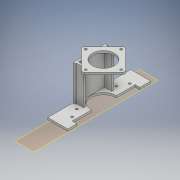
# Autodesk Inventor part: BAseSupport
Saved by Autodesk Inventor 2018 (Build 220112000, 112)
## iProperties
Created: 2017-08-08
Part Number: BAseSupport
Material: Generic
Document SubType Name: Modeling
Designer: M215104
Density: 1 g/cm^3
Appearance: Default
Author: M215104
Autodesk Inventor part; units mm, degrees
ref_plane "YZ Plane" through (0, 0, 0) normal (1, 0, 0) x (0, 1, 0)
ref_plane "XZ Plane" through (0, 0, 0) normal (0, 1, 0) x (-1, 0, 0)
ref_plane "XY Plane" through (0, 0, 0) normal (0, 0, 1) x (1, 0, 0)
ref_plane "Work Plane1" through (0, 2.2013, 0) normal (0, 0, 1) x (1, 0, 0)
sketch "Sketch1" plane through (0, 2.2013, 0) normal (0, 0, 1) x (1, 0, 0)
  arc A0 (50.7, -89.2086) -> (50.7, -149.194) centre (33.15, -119.2013) ccw construction
  circle A1 centre (30.5, -119.2013) radius 14.9 construction
  line L0 (34, -32.2013) -> (47, -32.2013) projected
  line L1 (47, -2.2013) -> (47, -32.2013) construction
  line L2 (0, -2.2013) -> (47, -2.2013) construction
  line L3 (0, -2.2013) -> (0, -315.2013) construction
  line L4 (0, -315.2013) -> (47, -315.2013) construction
  line L5 (47, -207.2013) -> (47, -315.2013) construction
  line L6 (47, -207.2013) -> (34, -207.2013) projected
  line L7 (34, -207.2013) -> (34, -193.2013) construction
  line L8 (34, -193.2013) -> (36, -193.2013) construction
  line L9 (36, -193.2013) -> (36, -155.499) construction
  line L10 (36, -155.499) -> (47, -163.2013) construction
  line L11 (47, -67.2013) -> (47, -163.2013) construction
  line L12 (47, -67.2013) -> (36, -74.9036) construction
  line L13 (36, -74.9036) -> (36, -45.2013) construction
  line L14 (36, -45.2013) -> (34, -45.2013) construction
  line L15 (34, -45.2013) -> (34, -32.2013) construction
  line L16 (47, -32.2013) -> (47, -2.2013)
  line L17 (47, -2.2013) -> (-8, -2.2013)
  line L18 (-8, -2.2013) -> (-8, -232.2013)
  line L19 (-8, -232.2013) -> (47, -232.2013)
  line L20 (47, -207.2013) -> (34, -207.2013) construction
  line L21 (34, -32.2013) -> (47, -32.2013) construction
  line L22 (47, -232.2013) -> (47, -207.2013)
  line L23 (47, -32.2013) -> (34, -32.2013)
  arc A2 (34, -84.4617) -> (34, -153.9409) centre (33.15, -119.2013) ccw
  line L24 (34, -207.2013) -> (34, -153.9409)
  line L25 (34, -84.4617) -> (34, -32.2013)
  dimension "d0" = 55
  dimension "d1" = 230
  constraints: 20 end point, 5 collinear, 2 parallel, 2 perpendicular, 2 point on circle, 2 point on line, 1 centre point, 1 coincident, 1 concentric
  measures "d0" distance of L1.start L17.end
  measures "d1" distance of L17.end L18.end
extrude "Extrusion1" add sketch "Sketch1" along normal blind 6
sketch "Sketch2" plane through (0, 2.2013, 6) normal (0, 0, 1) x (1, 0, 0)
  line L0 (-8, -2.2013) -> (-8, -232.2013) projected
  line L1 (-8, -117.2013) -> (-2, -117.2013)
  line L2 (-2, -117.2013) -> (-2, -162.2013)
  line L3 (-2, -162.2013) -> (-8, -162.2013)
  line L4 (-8, -162.2013) -> (-8, -117.2013)
  line L5 (-2, -117.2013) -> (-2, -72.2013)
  line L6 (-2, -72.2013) -> (-8, -72.2013)
  line L7 (-8, -72.2013) -> (-8, -117.2013)
  point P0 (0, -2.2013)
  dimension "d4" = 6
  dimension "d5" = 45
  constraints: 14 end point, 2 parallel, 2 symmetric about line, 1 horizontal, 1 midpoint, 1 perpendicular
  measures "d4" distance of L2.end L3.end
  measures "d5" distance of L1.end L2.end
extrude "Extrusion2" add sketch "Sketch2" along normal blind 97.5
sketch "Sketch3" plane through (0, 2.2013, 103.5) normal (0, 0, 1) x (1, 0, 0)
  line L0 (34, -207.2013) -> (34, -153.9409) construction
  line L1 (-27.6612, -119.2013) -> (33.15, -58.3901)
  line L2 (33.15, -58.3901) -> (93.9612, -119.2013)
  line L3 (93.9612, -119.2013) -> (33.15, -180.0125)
  line L4 (33.15, -180.0125) -> (-27.6612, -119.2013)
  arc A0 (34, -84.4617) -> (34, -153.9409) centre (33.15, -119.2013) ccw construction
  line L5 (-9.85, -76.2013) -> (76.15, -162.2013) construction
  line L6 (76.15, -76.2013) -> (-9.85, -162.2013) construction
  line L7 (-8, -162.2013) -> (-2, -162.2013) projected
  line L8 (-2, -162.2013) -> (15.3388, -162.2013)
  line L9 (-2, -162.2013) -> (-2, -72.2013) projected
  line L10 (-2, -72.2013) -> (19.3388, -72.2013)
  point P0 (0, -2.2013)
  point P1 (33.15, -117)
  dimension "d8" = 86
  dimension "d9" = 86
  constraints: 16 end point, 2 midpoint, 2 parallel, 2 point on line, 1 collinear, 1 horizontal, 1 perpendicular, 1 other
  measures "d8" distance of L2.end L3.end
  measures "d9" distance of L1.end L2.end
extrude "Extrusion3" add sketch "Sketch3" along normal blind 6 contours L1 L2 L3 L4 L9 | L9 L4 L1
sketch "Sketch4" plane through (0, 2.2013, 109.5) normal (0, 0, 1) x (1, 0, 0)
  arc A0 (34, -84.4617) -> (34, -153.9409) centre (33.15, -119.2013) ccw projected
  circle A1 centre (33.15, -119.2013) radius 30.5
  point P0 (0, -2.2013)
  dimension "d12" = 61
  constraints: 1 centre point, 1 coincident
  measures "d12" diameter of A1
extrude "Extrusion4" cut sketch "Sketch4" against normal blind 6
sketch "Sketch5" plane through (0, 2.2013, 6) normal (0, 0, 1) x (1, 0, 0)
  line L0 (-2, -72.2013) -> (-2, -162.2013) projected
  circle A0 centre (33.15, -119.2013) radius 30.5 projected
  circle A1 centre (33.15, -119.2013) radius 30.5 projected
  line L1 (33.15, -58.3901) -> (-27.6612, -119.2013) projected
  line L2 (-27.6612, -119.2013) -> (33.15, -180.0125) projected
  line L3 (33.15, -180.0125) -> (93.9612, -119.2013) projected
  line L4 (93.9612, -119.2013) -> (33.15, -58.3901) projected
  line L5 (-2, -75) -> (18, -75)
  line L6 (18, -75) -> (18, -81)
  line L7 (18, -81) -> (-2, -81)
  line L8 (-2, -81) -> (-2, -75)
  line L9 (-2, -117.2013) -> (14.539, -117.2013) construction
  line L10 (-8, -2.2013) -> (-8, -232.2013) projected
  line L11 (-2, -159.4026) -> (18, -159.4026)
  line L12 (18, -159.4026) -> (18, -153.4026)
  line L13 (18, -153.4026) -> (-2, -153.4026)
  line L14 (-2, -153.4026) -> (-2, -159.4026)
  point P0 (0, -2.2013)
  dimension "d15" = 20
  dimension "d16" = 6
  constraints: 18 end point, 4 symmetric about line, 2 parallel, 2 perpendicular, 1 horizontal, 1 midpoint, 1 point on line
  measures "d15" distance of L6.end L7.end
  measures "d16" distance of L5.end L6.end
extrude "Extrusion5" add sketch "Sketch5" along normal blind 97.5 contours L5 L1 L7 L0 | L5 L6 L7 L1 | L13 L2 L11 L0 | L13 L12 L11 L2
sketch "Sketch8" plane through (0, 2.2013, 103.5) normal (0, 0, -1) x (-1, 0, 0)
  circle A0 centre (-82.3646, -119.2013) radius 3.25 projected
  circle A1 centre (-82.3646, -119.2013) radius 3.25 projected
  circle A2 centre (-82.3646, -119.2013) radius 3.25 projected
  circle A3 centre (-82.3646, -119.2013) radius 3.25 projected
  circle A4 centre (-82.3646, -119.2013) radius 3.25 projected
  circle A5 centre (-82.3646, -119.2013) radius 3.25 projected
  circle A6 centre (-82.3646, -119.2013) radius 3.25 projected
  circle A7 centre (-82.3646, -119.2013) radius 3.25 projected
  circle A8 centre (-82.3646, -119.2013) radius 3.25 projected
  circle A9 centre (-82.3646, -119.2013) radius 3.25 projected
  circle A10 centre (-33.15, -69.9867) radius 3.25 projected
  circle A11 centre (16.0646, -119.2013) radius 3.25 projected
  circle A12 centre (-33.15, -168.4159) radius 3.25 projected
  point P0 (0, -2.2013)
extrude "Extrusion8" cut sketch "Sketch8" against normal blind 6
fillet "Fillet1" radius 5 4 edges at (93.9612, -117, 106.5) (33.15, -56.1888, 106.5) (-27.6612, -117, 106.5) (33.15, -177.8112, 106.5)
sketch "Sketch9" plane through (0, 2.2013, 6) normal (0, 0, 1) x (1, 0, 0)
  line L0 (-8, -2.2013) -> (-8, -232.2013) construction
  line L1 (-8, -117.2013) -> (28.1945, -117.2013) construction
  line L2 (34, -84.4617) -> (34, -32.2013) projected
  line L3 (34, -42.4176) -> (46, -42.4176) construction
  circle A0 centre (24, -37.2013) radius 3
  line L4 (0.6123, -2.2013) -> (0.6123, -307.2013) construction
  line L5 (47, -2.2013) -> (-8, -2.2013) projected
  circle A1 centre (12, -62.2013) radius 3
  circle A2 centre (24, -197.2013) radius 3
  circle A3 centre (12, -172.2013) radius 3
  point P0 (0, -2.2013)
  dimension "d32" = 6
  dimension "d36" = 10
  dimension "d37" = 35
  dimension "d40" = 6
  dimension "d44" = 20
  dimension "d45" = 25
  constraints: 4 centre point, 4 end point, 2 horizontal, 2 symmetric about line, 1 midpoint, 1 point on line, 2 other
  measures "d32" diameter of A0
  measures "d36" distance from line of L2 A0.centre
  measures "d37" distance from line of L5 A0.centre
  measures "d40" diameter of A1
  measures "d44" distance from line of L0 A1.centre
  measures "d45" vertical distance of A0.centre A1.centre
extrude "Extrusion9" cut sketch "Sketch9" against normal blind 6
body "Solid1"
